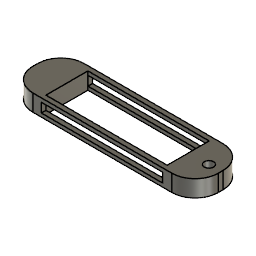
ARM_TOP (Assembly) (Autodesk Fusion 360 archive; units mm, degrees)
design "ARM_MID"
Autodesk Fusion 360 part; units mm, degrees
sketch "Sketch1" plane through (0, 0, 0) normal (0, 0, 1) x (1, 0, 0)
  line L0 (0, 0) -> (-200, 0)
  line L1 (-200, 0) -> (-200, 25)
  line L2 (-200, 25) -> (0, 25)
  line L3 (0, 25) -> (0, 0)
  constraint horizontal L0
  constraint vertical L1
  constraint horizontal L2
  constraint vertical L3
  constraint coincident L0.start L3.end
extrude "Extrude1" add sketch "Sketch1" along normal blind 30
ref_plane "WorkPlane2" through (-100, 12.5, 15) normal (1, 0, 0) x (0, 1, 0)
sketch "Sketch2" plane through (0, 0, 0) normal (0, -1, 0) x (1, 0, 0)
  line L0 (-200, 0) -> (0, 0)
  line L1 (0, 0) -> (0, 30)
  line L2 (0, 30) -> (-200, 30)
  line L3 (-200, 30) -> (-200, 0)
ref_plane "WorkPlane1" through (-100, 12.5, 15) normal (0, 0, 1) x (1, 0, 0)
sketch "Sketch3" plane through (0, 0, 15) normal (0, 0, 1) x (1, 0, 0)
  line L0 (-200, 25) -> (-180, 25)
  line L1 (-180, 25) -> (-180, 0)
  line L2 (-180, 0) -> (-200, 0)
  line L3 (-200, 0) -> (-200, 25)
  constraint horizontal L0
  constraint vertical L1
  constraint horizontal L2
  constraint vertical L3
extrude "Extrude2" cut 1 faces at (-200, 8.3333, 20) along direction (1, 0, 0) blind 1
sketch "Sketch4" plane through (0, 0, 30) normal (0, 0, 1) x (-1, 0, 0)
  line L0 (0, -25) -> (199, -25)
  line L1 (199, 0) -> (0, 0)
  line L2 (0, 0) -> (22, 0)
  line L3 (22, 0) -> (22, -25)
  line L4 (22, -25) -> (0, -25)
  line L5 (0, -25) -> (0, 0)
  line L6 (199, -25) -> (199, 0)
  line L7 (0, 0) -> (0, -25)
  constraint horizontal L2
  constraint vertical L3
  constraint horizontal L4
  constraint vertical L5
  constraint coincident L0 L3.end
  constraint coincident L1.end L2.start
extrude "Extrude3" cut sketch "Sketch4" against normal blind 6 contours L0 L1 L2 L3 L4 L5 L7
sketch "Sketch5" plane through (0, 0, 0) normal (0, 0, -1) x (1, 0, 0)
  line L0 (0, 0) -> (-199, 0)
  line L1 (-199, -25) -> (0, -25)
  line L2 (0, 0) -> (-22, 0)
  line L3 (-22, 0) -> (-22, -25)
  line L4 (-22, -25) -> (0, -25)
  line L5 (0, -25) -> (0, 0)
  line L6 (-199, 0) -> (-199, -25)
  line L7 (0, -25) -> (0, 0)
  constraint horizontal L2
  constraint vertical L3
  constraint horizontal L4
  constraint vertical L5
  constraint coincident L0.start L2.start
extrude "Extrude4" cut sketch "Sketch5" against normal blind 6 contours L0 L1 L2 L3 L4 L5 L7
sketch "Sketch6" plane through (0, 0, 30) normal (0, 0, 1) x (-1, 0, 0)
  line L0 (199, 0) -> (22, 0)
  line L1 (22, 0) -> (22, -25)
  line L2 (22, -25) -> (199, -25)
  line L3 (34.9313, -5) -> (165.0687, -5)
  line L4 (165.0687, -5) -> (165.0687, -20)
  line L5 (165.0687, -20) -> (34.9313, -20)
  line L6 (34.9313, -20) -> (34.9313, -5)
  line L7 (199, -25) -> (199, 0)
  constraint horizontal L3
  constraint vertical L4
  constraint horizontal L5
  constraint vertical L6
extrude "Extrude5" cut sketch "Sketch6" against normal blind 43 contours L3 L4 L5 L6
sketch "Sketch7" plane through (0, 25, 0) normal (0, 1, 0) x (-1, 0, 0)
  line L0 (199, 30) -> (22, 30)
  line L1 (22, 30) -> (22, 24)
  line L2 (22, 24) -> (0, 24)
  line L3 (0, 6) -> (22, 6)
  line L4 (22, 6) -> (22, 0)
  line L5 (22, 0) -> (199, 0)
  line L6 (34.8715, 24.9016) -> (165.0188, 24.9016)
  line L7 (165.0188, 24.9016) -> (165.0188, 4.9016)
  line L8 (165.0188, 4.9016) -> (34.8715, 4.9016)
  line L9 (34.8715, 4.9016) -> (34.8715, 24.9016)
  line L10 (199, 0) -> (199, 30)
  line L11 (0, 24) -> (0, 6)
  dimension "d20" = 20
  constraint horizontal L6
  constraint vertical L7
  constraint horizontal L8
  constraint vertical L9
  measures "d20" distance of L6.start L8.end
extrude "Extrude6" cut sketch "Sketch7" against normal blind 50 contours L6 L7 L8 L9
sketch "Sketch8" plane through (0, 25, 0) normal (0, 1, 0) x (-1, 0, 0)
sketch "Sketch9" plane through (0, 0, 30) normal (0, 0, 1) x (-1, 0, 0)
  line L0 (165.0687, -5) -> (165.0687, -20)
  line L1 (165.0687, -20) -> (34.9313, -20)
  line L2 (34.9313, -20) -> (34.9313, -5)
  line L3 (34.9313, -5) -> (165.0687, -5)
  line L4 (199, 0) -> (22, 0)
  line L5 (22, 0) -> (22, -25)
  line L6 (22, -25) -> (199, -25)
  line L7 (22, -17.5) -> (37.5, -25)
  line L8 (22, -25) -> (37.5, -25)
  line L9 (22, -25) -> (22, -17.5)
  line L10 (199, -25) -> (199, 0)
  constraint coincident L5 L7.start
  constraint coincident L6 L7.end
  constraint coincident L5.end L6.start
ref_plane "WorkPlane3" through (-99.5, 12.5, 15) normal (0, 1, 0) x (-1, 0, 0)
sketch "Sketch10" plane through (0, 0, 30) normal (0, 0, 1) x (-1, 0, 0)
extrude "Extrude7" add 1 faces at (-78.2739, 1.6667, 24.9016) along direction (0, 0, -1) blind 5
extrude "Extrude8" add 1 faces at (-78.2739, 1.6667, 4.9016) along direction (0, 0, 1) blind 5
sketch "Sketch11" plane through (-22, 0, 0) normal (1, 0, 0) x (0, 1, 0)
  line L0 (25, 30) -> (0, 30)
  line L1 (0, 30) -> (0, 24)
  line L2 (0, 24) -> (25, 24)
  line L3 (25, 24) -> (25, 30)
  line L4 (0, 30) -> (25, 30)
  line L5 (25, 30) -> (25, 24)
  line L6 (25, 24) -> (0, 24)
  line L7 (0, 24) -> (0, 30)
  line L8 (0, 6) -> (25, 6)
  line L9 (25, 6) -> (25, 0)
  line L10 (25, 0) -> (0, 0)
  line L11 (0, 0) -> (0, 6)
  constraint horizontal L4
  constraint vertical L5
  constraint horizontal L6
  constraint vertical L7
  constraint coincident L2.end L3.start
  constraint coincident L0.end L1.start
  constraint horizontal L8
  constraint vertical L9
  constraint horizontal L10
  constraint vertical L11
extrude "Extrude9" cut sketch "Sketch11" against normal blind 220
sketch "Sketch12" plane through (0, 0, 24) normal (0, 0, 1) x (-1, 0, 0)
  line L0 (34.9313, -5) -> (165.0687, -5)
  line L1 (165.0687, -5) -> (165.0687, -20)
  line L2 (165.0687, -20) -> (34.9313, -20)
  line L3 (34.9313, -20) -> (34.9313, -5)
  line L4 (0, -25) -> (199, -25)
  line L5 (199, 0) -> (0, 0)
  line L6 (25, -25) -> (25, 0)
  line L7 (199, -25) -> (199, 0)
  line L8 (0, 0) -> (0, -25)
  constraint vertical L6
extrude "Extrude10" add 1 faces at (-187.6729, 0, 16.6339) along direction (0, -1, 0) blind 30
sketch "Sketch13" plane through (0, 0, 24) normal (0, 0, 1) x (-1, 0, 0)
  line L0 (34.9313, -5) -> (165.0687, -5)
  line L1 (165.0687, -5) -> (165.0687, -20)
  line L2 (165.0687, -20) -> (34.9313, -20)
  line L3 (34.9313, -20) -> (34.9313, -5)
  line L4 (0, -25) -> (199, -25)
  line L5 (199, 30) -> (0, 30)
  line L6 (165, -5) -> (35, -5)
  line L7 (35, -5) -> (35, 25)
  line L8 (35, 25) -> (165, 25)
  line L9 (165, 25) -> (165, -5)
  line L10 (35, -5) -> (165, -5)
  line L11 (165, -5) -> (165, 25)
  line L12 (165, 25) -> (35, 25)
  line L13 (35, 25) -> (35, -5)
  line L14 (199, -25) -> (199, 30)
  line L15 (0, 30) -> (0, -25)
  constraint horizontal L6
  constraint vertical L7
  constraint horizontal L8
  constraint vertical L9
  constraint horizontal L10
  constraint vertical L11
  constraint horizontal L12
  constraint vertical L13
sketch "Sketch14" plane through (0, 0, 24) normal (0, 0, 1) x (-1, 0, 0)
  line L0 (34.9313, -5) -> (165.0687, -5)
  line L1 (165.0687, -5) -> (165.0687, -20)
  line L2 (165.0687, -20) -> (34.9313, -20)
  line L3 (34.9313, -20) -> (34.9313, -5)
  line L4 (0, -25) -> (199, -25)
  line L5 (199, 30) -> (0, 30)
  line L6 (165, -5) -> (35, -5)
  line L7 (35, -5) -> (35, 25)
  line L8 (35, 25) -> (165, 25)
  line L9 (165, 25) -> (165, -5)
  line L10 (35, 25) -> (165, 25)
  line L11 (165, 25) -> (165, -5)
  line L12 (165, -5) -> (35, -5)
  line L13 (35, -5) -> (35, 25)
  line L14 (199, -25) -> (199, 30)
  line L15 (0, 30) -> (0, -25)
  constraint horizontal L6
  constraint vertical L7
  constraint horizontal L8
  constraint vertical L9
  constraint horizontal L10
  constraint vertical L11
  constraint horizontal L12
  constraint vertical L13
extrude "Extrude11" cut 1 faces at (-121.6729, 5, 22.6339) along direction (0, -1, 0) blind 30
fillet "Fillet3" radius 25 2 edges at (0, 25, 15) (0, -30, 15)
fillet "Fillet4" radius 25 2 edges at (-199, 25, 15) (-199, -30, 15)
hole "Hole2" at (-13.2303, -1.87, 24) direction (0, 0, -1) diameter 10 depth 40 tip angle 118
scale "Scale1" factor 0.7 about (-34.9313, 20, 24) bodies 1

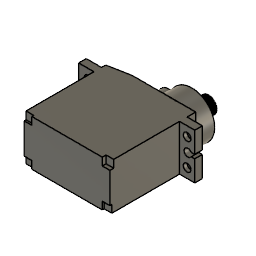
design "motor"
Autodesk Fusion 360 part; units mm, degrees
sketch "Sketch1" plane through (0, 0, 0) normal (0, 0, 1) x (1, 0, 0)
  line L0 (0, 0) -> (22.5, 0)
  line L1 (22.5, 0) -> (22.5, 22.5)
  line L2 (22.5, 22.5) -> (0, 22.5)
  line L3 (0, 22.5) -> (0, 0)
  dimension "d1" = 22.5
  dimension "d2" = 22.5
  constraint horizontal L0
  constraint vertical L1
  constraint horizontal L2
  constraint vertical L3
  constraint coincident L0.start L3.end
  measures "d1" distance of L0.start L0.end
  measures "d2" distance of L0.start L2.end
extrude "Extrude1" add sketch "Sketch1" along normal blind 12
sketch "Sketch2" plane through (0, 0, 0) normal (0, 0, 1) x (1, 0, 0)
  line L0 (24, 0) -> (24, 18.3) construction
  dimension "d5" = 18.3
  constraint vertical L0
  measures "d5" distance of L0.start L0.end
sketch "Sketch3" plane through (22.5, 0, 0) normal (1, 0, 0) x (0, 1, 0)
  line L0 (0, 0) -> (22.5, 0)
  line L1 (22.5, 0) -> (22.5, 12)
  line L2 (22.5, 12) -> (0, 12)
  line L3 (0, 12) -> (0, 0)
  line L4 (18.2502, 0) -> (20.2502, 0)
  line L5 (20.2502, 0) -> (20.2502, 12)
  line L6 (20.2502, 12) -> (18.2502, 12)
  line L7 (18.2502, 12) -> (18.2502, 0)
  dimension "d6" = 2
  constraint horizontal L4
  constraint vertical L5
  constraint horizontal L6
  constraint vertical L7
  constraint coincident L0 L4.start
  measures "d6" distance of L4.start L4.end
extrude "Extrude2" add sketch "Sketch3" along normal blind 4 contours L0 L2 L4 L5 L6 L7
sketch "Sketch4" plane through (0, 0, 0) normal (-1, 0, 0) x (0, -1, 0)
  line L0 (-22.5, 0) -> (0, 0)
  line L1 (0, 0) -> (0, 12)
  line L2 (0, 12) -> (-22.5, 12)
  line L3 (-22.5, 12) -> (-22.5, 0)
  line L4 (-18.3, 0) -> (-20.3, 0)
  line L5 (-20.3, 0) -> (-20.3, 12)
  line L6 (-20.3, 12) -> (-18.3, 12)
  line L7 (-18.3, 12) -> (-18.3, 0)
  dimension "d9" = 2
  dimension "d10" = 12
  constraint horizontal L4
  constraint vertical L5
  constraint horizontal L6
  constraint vertical L7
  constraint coincident L0 L4.start
  measures "d9" distance of L4.start L4.end
  measures "d10" distance of L4.start L6.end
extrude "Extrude3" add sketch "Sketch4" along normal blind 4 contours L0 L2 L4 L5 L6 L7
sketch "Sketch5" plane through (0, 20.2502, 0) normal (0, 1, 0) x (-1, 0, 0)
  line L0 (-22.5, 0) -> (-22.5, 12)
  line L1 (-22.5, 12) -> (-26.5, 12)
  line L2 (-26.5, 12) -> (-26.5, 0)
  line L3 (-26.5, 0) -> (-22.5, 0)
  line L4 (-26.5, 6) -> (-24.7, 6) construction
  circle A0 centre (-24.7, 6) radius 1
  line L5 (-24.7, 6) -> (7.4246, 6) construction
  line L6 (4, 6) -> (2.2, 6) construction
  circle A1 centre (2.2, 6) radius 1
  dimension "d13" = 1.8
  dimension "d14" = 2
  dimension "d15" = 1.8
  dimension "d16" = 2
  constraint midpoint L2 L4.start
  constraint perpendicular L2 L4
  constraint coincident L4.end A0.centre
  constraint perpendicular L2 L5
  constraint coincident L5 L6.start
  constraint parallel L5 L6
  constraint coincident L6.end A1.centre
  measures "d13" distance of L4.start L4.end
  measures "d14" diameter of A0
  measures "d15" distance of L6.start L6.end
  measures "d16" diameter of A1
extrude "Extrude4" cut sketch "Sketch5" against normal blind 2 contours A0
sketch "Sketch6" plane through (0, 20.3, 0) normal (0, 1, 0) x (-1, 0, 0)
  line L0 (0, 12) -> (0, 0)
  line L1 (0, 0) -> (4, 0)
  line L2 (4, 0) -> (4, 12)
  line L3 (4, 12) -> (0, 12)
  line L4 (4, 6) -> (2.2, 6)
  circle A0 centre (2.2, 6) radius 1
  dimension "d19" = 1.8
  dimension "d20" = 2
  constraint midpoint L2 L4.start
  constraint perpendicular L2 L4
  constraint coincident L4.end A0.centre
  measures "d19" distance of L4.start L4.end
  measures "d20" diameter of A0
extrude "Extrude5" cut sketch "Sketch6" against normal blind 2 contours A0
sketch "Sketch7" plane through (0, 20.3, 0) normal (0, 1, 0) x (-1, 0, 0)
  circle A0 centre (2.2, 6) radius 1
  line L0 (0, 12) -> (0, 0)
  line L1 (0, 0) -> (4, 0)
  line L2 (4, 0) -> (4, 12)
  line L3 (4, 12) -> (0, 12)
  line L4 (2.7402, 6.5) -> (5.2598, 6.5)
  line L5 (5.2598, 6.5) -> (5.2598, 5.5)
  line L6 (5.2598, 5.5) -> (2.7402, 5.5)
  line L7 (2.7402, 5.5) -> (2.7402, 6.5)
  line L8 (2.7402, 6.5) -> (5.2598, 5.5) construction
  line L9 (5.2598, 6.5) -> (2.7402, 5.5) construction
  point P0 (4, 6)
  dimension "d23" = 1
  constraint horizontal L4
  constraint perpendicular L4 L5
  constraint parallel L4 L6
  constraint parallel L5 L7
  constraint coincident L8 P0
  constraint coincident L9 P0
  constraint midpoint L2 P0
  measures "d23" distance of L4.end L5.end
extrude "Extrude6" cut sketch "Sketch7" against normal blind 2 contours A0 L2 L4 L6
sketch "Sketch8" plane through (0, 20.2502, 0) normal (0, 1, 0) x (-1, 0, 0)
  circle A0 centre (-24.7, 6) radius 1
  line L0 (-22.5, 0) -> (-22.5, 12)
  line L1 (-22.5, 12) -> (-26.5, 12)
  line L2 (-26.5, 12) -> (-26.5, 0)
  line L3 (-26.5, 0) -> (-22.5, 0)
  line L4 (-25.5, 5.5) -> (-27.5, 5.5)
  line L5 (-27.5, 5.5) -> (-27.5, 6.5)
  line L6 (-27.5, 6.5) -> (-25.5, 6.5)
  line L7 (-25.5, 6.5) -> (-25.5, 5.5)
  line L8 (-25.5, 5.5) -> (-27.5, 6.5) construction
  line L9 (-27.5, 5.5) -> (-25.5, 6.5) construction
  point P0 (-26.5, 6)
  constraint horizontal L4
  constraint perpendicular L4 L5
  constraint parallel L4 L6
  constraint parallel L5 L7
  constraint coincident L8 P0
  constraint coincident L9 P0
  constraint midpoint L2 P0
extrude "Extrude7" cut sketch "Sketch8" against normal blind 2 contours A0 L2 L4 L6
sketch "Sketch9" plane through (0, 22.5, 0) normal (0, 1, 0) x (-1, 0, 0)
  line L0 (-22.5, 0) -> (0, 0)
  line L1 (0, 0) -> (0, 12)
  line L2 (0, 12) -> (-22.5, 12)
  line L3 (-22.5, 12) -> (-22.5, 0)
  line L4 (0, 6) -> (-7.7, 6) construction
  circle A0 centre (-10.45, 6) radius 2.75
  circle A1 centre (-16.5, 6) radius 6
  dimension "d28" = 7.7
  dimension "d29" = 5.5
  dimension "d30" = 12
  constraint midpoint L1 L4.start
  constraint perpendicular L1 L4
  constraint coincident L4.end A0
  measures "d28" distance of L4.start L4.end
  measures "d29" diameter of A0
  measures "d30" diameter of A1
extrude "Extrude8" add sketch "Sketch9" along normal blind 5 contours A0 A1 | A0 A1 | A0 A1
sketch "Sketch10" plane through (0, 0, 0) normal (0, 0, -1) x (1, 0, 0)
  line L0 (0, -20.3) -> (0, -22.5)
  line L1 (0, -22.5) -> (16.5, -22.5)
  line L2 (16.5, -22.5) -> (22.5, -22.5)
  line L3 (22.5, -22.5) -> (22.5, -20.2502)
  line L4 (22.5, -20.2502) -> (26.5, -20.2502)
  line L5 (26.5, -20.2502) -> (26.5, -18.2502)
  line L6 (26.5, -18.2502) -> (22.5, -18.2502)
  line L7 (22.5, -18.2502) -> (22.5, 0)
  line L8 (22.5, 0) -> (0, 0)
  line L9 (0, 0) -> (0, -18.3)
  line L10 (0, -18.3) -> (-4, -18.3)
  line L11 (-4, -18.3) -> (-4, -20.3)
  line L12 (-4, -20.3) -> (0, -20.3)
  line L13 (0, -22.5) -> (0, -21.4) construction
  line L14 (0, -21.4) -> (5.8985, -22.4988)
  line L15 (0, -21.4) -> (0, -22.5)
  line L16 (0, -22.5) -> (5.8985, -22.4988)
  dimension "d33" = 1.1
  dimension "d34" = 6
  constraint coincident L0.end L1.start
  constraint perpendicular L1 L13
  measures "d33" distance of L0.end L13.end
  measures "d34" distance of L13.end L14.end
extrude "Extrude9" cut sketch "Sketch10" against normal blind 12 contours L0 L14 L15 L16
sketch "Sketch11" plane through (0, 22.5, 0) normal (0, 1, 0) x (-1, 0, 0)
  arc A0 (-11.1248, 8.6659) -> (-16.5, 12) centre (-16.5, 6) ccw
  arc A1 (-11.1248, 3.3341) -> (-11.1248, 8.6659) centre (-10.45, 6) ccw
  arc A2 (-16.5, 0) -> (-11.1248, 3.3341) centre (-16.5, 6) ccw
  line L0 (-16.5, 0) -> (0, 0)
  line L1 (0, 0) -> (0, 12)
  line L2 (0, 12) -> (-16.5, 12)
  line L3 (0, 0) -> (-5.9, 0)
  line L4 (-5.9, 0) -> (-5.9, 12)
  line L5 (-5.9, 12) -> (0, 12)
  line L6 (0, 12) -> (0, 0)
  constraint horizontal L3
  constraint vertical L4
  constraint horizontal L5
  constraint vertical L6
  constraint coincident L2 L4.end
  constraint coincident L0.end L1.start
extrude "Extrude10" cut sketch "Sketch11" against normal blind 0.002 contours L0 L1 L2 L3 L4 L5 L6
sketch "Sketch12" plane through (0, 0, 0) normal (0, -1, 0) x (1, 0, 0)
  line L0 (0, 0) -> (22.5, 0)
  line L1 (22.5, 0) -> (22.5, 12)
  line L2 (22.5, 12) -> (0, 12)
  line L3 (0, 12) -> (0, 0)
  line L4 (22.5, 6) -> (20.8, 6)
  line L5 (22.5, 3.65) -> (20.8, 3.65)
  line L6 (20.8, 3.65) -> (20.8, 8.35)
  line L7 (20.8, 8.35) -> (22.5, 8.35)
  line L8 (22.5, 8.35) -> (22.5, 3.65)
  line L9 (22.5, 3.65) -> (20.8, 8.35) construction
  line L10 (20.8, 3.65) -> (22.5, 8.35) construction
  point P0 (21.65, 6)
  dimension "d39" = 1.7
  dimension "d40" = 4.7
  constraint midpoint L1 L4.start
  constraint perpendicular L1 L4
  constraint horizontal L5
  constraint perpendicular L5 L6
  constraint parallel L5 L7
  constraint parallel L6 L8
  constraint coincident L9 P0
  constraint coincident L10 P0
  constraint midpoint L4 P0
  measures "d39" distance of L4.start L4.end
  measures "d40" distance of L5.end L6.end
extrude "Extrude11" cut sketch "Sketch12" against normal blind 1.7 contours L1 L4 L5 L6 L8 | L1 L4 L6 L7 L8
sketch "Sketch13" plane through (20.8, 0, 0) normal (1, 0, 0) x (0, 1, 0)
  line L0 (0, 8.35) -> (0, 3.65)
  line L1 (0, 3.65) -> (1.7, 3.65)
  line L2 (1.7, 3.65) -> (1.7, 8.35)
  line L3 (1.7, 8.35) -> (0, 8.35)
  line L4 (0.5096, 8.35) -> (1.7, 8.35)
  line L5 (1.7, 8.35) -> (1.7, 3.65)
  line L6 (1.7, 3.65) -> (0.5096, 3.65)
  line L7 (0.5096, 3.65) -> (0.5096, 8.35)
  constraint horizontal L4
  constraint vertical L5
  constraint horizontal L6
  constraint vertical L7
  constraint coincident L1.end L2.start
  constraint coincident L3 L4.start
extrude "Extrude12" cut sketch "Sketch13" against normal blind 2 contours L1 L2 L3 L4 L5 L6 L7
sketch "Sketch14" plane through (0, 1.7, 0) normal (0, -1, 0) x (1, 0, 0)
  line L0 (22.5, 8.35) -> (18.8, 8.35)
  line L1 (18.8, 8.35) -> (18.8, 3.65)
  line L2 (18.8, 3.65) -> (22.5, 3.65)
  line L3 (22.5, 3.65) -> (22.5, 8.35)
  line L4 (22.0206, 8.35) -> (20.7831, 8.35)
  line L5 (20.7831, 8.35) -> (20.7831, 3.65)
  line L6 (20.7831, 3.65) -> (22.0206, 3.65)
  line L7 (22.0206, 3.65) -> (22.0206, 8.35)
  constraint horizontal L4
  constraint vertical L5
  constraint horizontal L6
  constraint vertical L7
  constraint coincident L2 L5.end
  constraint coincident L0 L4.start
extrude "Extrude13" cut sketch "Sketch14" against normal blind 4 contours L0 L2 L4 L5 L6 L7
sketch "Sketch15" plane through (0, 27.5, 0) normal (0, 1, 0) x (-1, 0, 0)
  arc A0 (-11.1248, 3.3341) -> (-11.1248, 8.6659) centre (-10.45, 6) ccw
  arc A1 (-11.1248, 8.6659) -> (-11.1248, 3.3341) centre (-16.5, 6) ccw
  circle A2 centre (-16.5, 6) radius 3.5
  dimension "d48" = 7
  constraint concentric A1 A2
  measures "d48" diameter of A2
extrude "Extrude14" add sketch "Sketch15" along normal blind 0.5 contours A2
sketch "Sketch16" plane through (0, 28, 0) normal (0, 1, 0) x (-1, 0, 0)
  circle A0 centre (-16.5, 6) radius 3.5
  circle A1 centre (-16.5, 6) radius 2.15
  dimension "d51" = 4.3
  constraint concentric A0 A1
  measures "d51" diameter of A1
extrude "Extrude15" add sketch "Sketch16" along normal blind 4 contours A1
ref_plane "WorkPlane1" through (16.5, 30.1431, 3.85) normal (0, 0, -1) x (1, 0, 0)
sketch "Sketch17" plane through (0, 0, 3.85) normal (0, 0, -1) x (-1, 0, 0)
ref_plane "WorkPlane3" through (16.5, 30.4646, 5.85) normal (0, 0, -1) x (1, 0, 0)
sketch "Sketch18" plane through (0, 0, 5.85) normal (0, 0, -1) x (-1, 0, 0)
  line L0 (-14.3401, 28) -> (-14.8401, 28)
  line L1 (-14.8401, 28) -> (-14.8401, 29.7)
  line L2 (-14.8401, 29.7) -> (-14.3401, 29.7)
  line L3 (-14.3401, 29.7) -> (-14.3401, 28)
  dimension "d57" = 0.5
  dimension "d58" = 1.7
  constraint horizontal L0
  constraint vertical L1
  constraint horizontal L2
  constraint vertical L3
  measures "d57" distance of L0.start L0.end
  measures "d58" distance of L0.start L2.end
revolve "Revolve1" cut sketch "Sketch18" angle 360 about axis through (16.5, 28, 6) along (0, -1, 0)
sketch "Sketch19" plane through (0, 32, 0) normal (0, 1, 0) x (-1, 0, 0)
  circle A0 centre (-16.5, 6) radius 2.15
  line L0 (-16.4999, 7.7485) -> (-16.3965, 8.1475)
  line L1 (-16.6035, 8.1475) -> (-16.4999, 7.7485)
  constraint coincident A0 L1.start
  constraint coincident A0 L0.end
extrude "Extrude16" cut sketch "Sketch19" against normal blind 3 contours A0 L0 L1 picked at (-16.5, 8.016)
pattern_circular "C-Pattern1" count 50 over 360 about axis through (16.5, 28, 6) along (0, 1, 0) of "Extrude16"
sketch "Sketch20" plane through (0, 0, 0) normal (0, -1, 0) x (1, 0, 0)
  line L0 (20.8, 8.35) -> (22.5, 8.35)
  line L1 (22.5, 8.35) -> (22.5, 12)
  line L2 (22.5, 12) -> (0, 12)
  line L3 (0, 12) -> (0, 0)
  line L4 (0, 0) -> (22.5, 0)
  line L5 (22.5, 0) -> (22.5, 3.65)
  line L6 (22.5, 3.65) -> (20.8, 3.65)
  line L7 (20.8, 3.65) -> (20.8, 8.35)
  line L8 (22.5, 12) -> (20.5, 12)
  line L9 (20.5, 12) -> (20.5, 10)
  line L10 (20.5, 10) -> (22.5, 10)
  line L11 (22.5, 10) -> (22.5, 12)
  line L12 (11.25, 12) -> (11.25, -2) construction
  line L13 (0, 6) -> (30, 6) construction
  line L14 (20.5, 0) -> (20.5, 2)
  line L15 (20.5, 2) -> (22.5, 2)
  line L16 (22.5, 2) -> (22.5, 0)
  line L17 (22.5, 0) -> (20.5, 0)
  line L18 (2, 2) -> (0, 2)
  line L19 (2, 0) -> (2, 2)
  line L20 (0, 0) -> (2, 0)
  line L21 (0, 2) -> (0, 0)
  line L22 (2, 10) -> (0, 10)
  line L23 (2, 12) -> (2, 10)
  line L24 (0, 12) -> (2, 12)
  line L25 (0, 10) -> (0, 12)
  dimension "d64" = 2
  dimension "d65" = 2
  constraint horizontal L8
  constraint vertical L9
  constraint horizontal L10
  constraint vertical L11
  constraint coincident L1.end L2.start
  constraint midpoint L2 L12.start
  constraint perpendicular L2 L12
  constraint midpoint L3 L13.start
  constraint perpendicular L3 L13
  constraint symmetric L1.end L13 L4.end
  constraint symmetric L8.end L13 L14.start
  constraint symmetric L9.end L13 L14.end
  constraint symmetric L10.end L13 L15.end
  constraint symmetric L1.end L12 L2.end
  constraint symmetric L8.end L12 L23.start
  constraint symmetric L9.end L12 L22.start
  constraint symmetric L10.end L12 L22.end
  constraint symmetric L12 L14.start L19.start
  constraint symmetric L12 L14.end L18.start
  constraint symmetric L12 L15.end L18.end
  constraint symmetric L12 L4.end L3.end
  measures "d64" distance of L1.end L8.end
  measures "d65" distance of L1.end L10.end
extrude "Extrude17" cut sketch "Sketch20" against normal blind 1 contours L1 L2 L8 L9 L10 L11
extrude "Extrude18" cut sketch "Sketch20" against normal blind 0.5 contours L1 L2 L8 L9 L10 L11 | L4 L5 L14 L15 L16 L17 | L2 L3 L22 L23 L24 L25 | L3 L4 L18 L19 L20 L21
sketch "Sketch21" plane through (0, 18.2502, 0) normal (0, -1, 0) x (1, 0, 0)
  line L0 (26.5, 5.5) -> (25.566, 5.5)
  arc A0 (25.566, 6.5) -> (25.566, 5.5) centre (24.7, 6) ccw
  line L1 (25.566, 6.5) -> (26.5, 6.5)
  line L2 (26.5, 6.5) -> (26.5, 12)
  line L3 (26.5, 12) -> (22.5, 12)
  line L4 (22.5, 12) -> (22.5, 0)
  line L5 (22.5, 0) -> (26.5, 0)
  line L6 (26.5, 0) -> (26.5, 5.5)
  circle A1 centre (24.5, 2.5) radius 1
  circle A2 centre (24.5, 9.5) radius 1
  circle A3 centre (-1.5, 2.5) radius 1
  circle A4 centre (-1.5, 9.5) radius 1
  dimension "d70" = 2
  dimension "d71" = 2
  dimension "d72" = 2
  measures "d70" diameter of A1
  measures "d71" diameter of A2
  measures "d72" diameter of A3
extrude "Extrude19" cut sketch "Sketch21" against normal blind 1 contours A1 | A2 | A3 | A4
hole "Hole1" at (16.5, 32, 6) direction (0, -1, 0) diameter 3 depth 0.5 tip angle 118
ref_plane "WorkPlane4" through (20.8, 0, 6) normal (-0.707107, 0.707107, 0) x (0, 0, 1)
sketch "Sketch22" plane through (10.4, -10.4, 0) normal (-0.707107, 0.707107, 0) x (0, 0, 1)
  circle A0 centre (6.6874, 15.9981) radius 0.75
  circle A1 centre (5.3069, 16.0168) radius 0.75
  dimension "d81" = 1.5
  dimension "d82" = 1.5
  measures "d81" diameter of A0
  measures "d82" diameter of A1
extrude "Extrude22" add 1 faces at (21.6081, 3.0333, 3.65) along direction (0, 0, 1) blind 5
